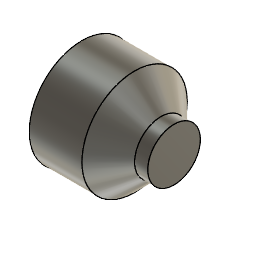
Part1 (Autodesk Fusion 360 design; units mm, degrees)
part number: 2026-06-25-05-00-46-965
Autodesk Fusion 360 part; units mm, degrees
sketch "Sketch1" plane through (0, 0, 0) normal (0, 0, 1) x (1, 0, 0)
  line L0 (0, 0) -> (0, 40)
  line L1 (0, 40) -> (40, 40)
  line L2 (40, 40) -> (60, 20)
  line L3 (60, 20) -> (70, 20)
  line L4 (70, 20) -> (70, 0)
  line L5 (70, 0) -> (0, 0)
  constraint coincident L0.start L5.end
  constraint vertical L0
  constraint perpendicular L0 L1
  constraint perpendicular L0 L3
  constraint perpendicular L3 L4
  constraint perpendicular L0 L5
revolve "Revolve1" add sketch "Sketch1" angle 360 about axis through (70, 0, 0) along (-1, 0, 0)
